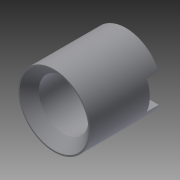
# Autodesk Inventor part: Cylindre
Saved by Autodesk Inventor 2014 SP2 (Build 180246200, 246)
## iProperties
Created: 2014-11-25
Part Number: Cylindre
Material: Générique
Document SubType Name: Modeling
Designer: sd
Density: 1 g/cm^3
Appearance: Par défaut
Author: sd
Autodesk Inventor part; units mm, degrees
ref_plane "YZ Plane" through (0, 0, 0) normal (1, 0, 0) x (0, 1, 0)
ref_plane "XZ Plane" through (0, 0, 0) normal (0, 1, 0) x (-1, 0, 0)
ref_plane "XY Plane" through (0, 0, 0) normal (0, 0, 1) x (1, 0, 0)
sketch "Esquisse1" plane through (0, 0, 0) normal (0, 1, 0) x (-1, 0, 0)
  ellipse E0 centre (0, 0) end of major axis (0, 15) minor radius 15
  dimension "d0" = 15
  dimension "d1" = 15
  constraints: 1 coincident, 2 other
extrude "Extrusion1" add sketch "Esquisse1" along normal blind 30
shell "Coque1" thickness 4.6 removed faces 1 at (0.1197, 0, 4.0636)
chamfer "Chanfrein1" distance 4 angle 45 1 edges at (-0.0005, 0, -10.4)
sketch "Esquisse3" plane through (0, 30, 0) normal (0, 1, 0) x (1, 0, 0)
  circle A0 centre (0, 0) radius 15 projected
  line L0 (-20, 6) -> (20, 6)
  line L1 (20, 6) -> (20, -6)
  line L2 (20, -6) -> (-20, -6)
  line L3 (-20, -6) -> (-20, 6)
  dimension "d14" = 12
  dimension "d15" = 6
  dimension "d16" = 40
  dimension "d17" = 20
  constraints: 8 end point, 2 parallel, 1 horizontal, 1 perpendicular
  measures "d14" distance of L2.end L0.start
  measures "d15" vertical distance of A0.centre L0.start
  measures "d16" distance of L0.start L0.end
  measures "d17" horizontal distance of A0.centre L0.start
extrude "Extrusion3" cut sketch "Esquisse3" against normal blind 5 contours A0 L2 L0 | A0 L0 L1 L2 | A0 L2 L3 L0
equation "\"d15\" = 0.5 * d14"
equation "\"d17\" = 0.5 * d16"
